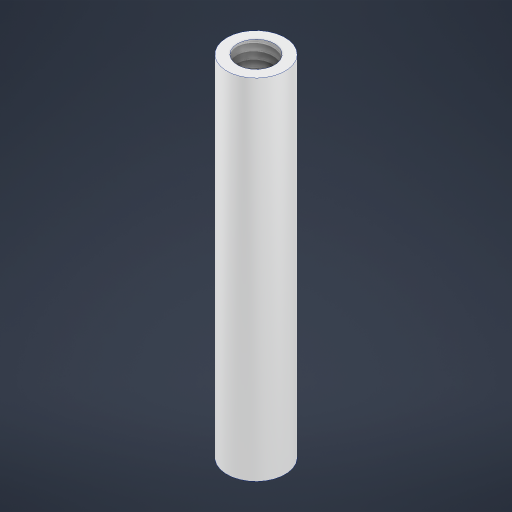
# Autodesk Inventor part: Gearboxes_003_standoff
Saved by Autodesk Inventor 2024.4 (Build 284460000, 460)
## iProperties
Created: 2026-06-11
Part Number: Gearboxes_003_standoff
Material: Aluminum 6061
Document SubType Name: Modeling
Designer: stanr
Density: 2.7 g/cm^3
Appearance: Aluminum - Flat
Author: stanr
Autodesk Inventor part; units mm, degrees
ref_plane "YZ Plane" through (0, 0, 0) normal (1, 0, 0) x (0, 1, 0)
ref_plane "XZ Plane" through (0, 0, 0) normal (0, 1, 0) x (-1, 0, 0)
ref_plane "XY Plane" through (0, 0, 0) normal (0, 0, 1) x (1, 0, 0)
sketch "Sketch1" plane through (0, 0, 0) normal (0, 1, 0) x (-1, 0, 0)
  circle A0 centre (0, 0) radius 3.175
  circle A1 centre (0, 0) radius 2.0193
  dimension "d0" = 6.35
  dimension "d1" = 4.0386
  constraints: 2 centre point, 2 coincident
  measures "d0" diameter of A0
  measures "d1" diameter of A1
extrude "Extrusion1" add sketch "Sketch1" along normal blind 38.1
thread "Thread1" size "10-32 UNF" class "2B" standard "ANSI Unified Screw Threads" full length
body "Solid1"
